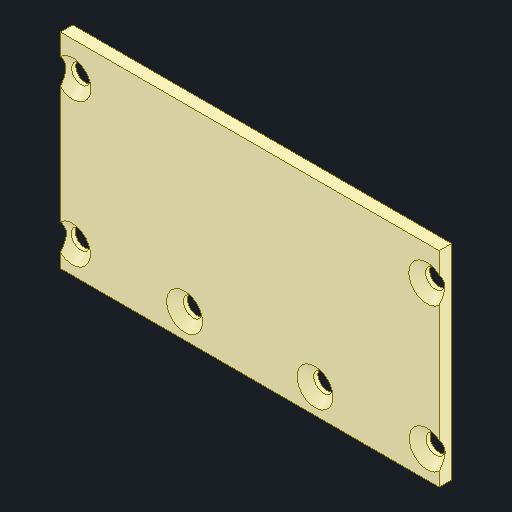
# Autodesk Inventor part: back
Saved by Autodesk Inventor 2023 (Build 270158000, 158)
## iProperties
Created: 2024-05-19
Part Number: back
Material: Nylon 6/6
Document SubType Name: Modeling
Designer: szymo
Density: 1.13 g/cm^3
Appearance: Nylon 6
Mass: 3.8512 g
Surface Area: 47.3773 cm^2
Volume: 3.40814 cm^3
Author: szymo
Autodesk Inventor part; units mm, degrees
ref_plane "YZ Plane" through (0, 0, 0) normal (1, 0, 0) x (0, 1, 0)
ref_plane "XZ Plane" through (0, 0, 0) normal (0, 1, 0) x (-1, 0, 0)
ref_plane "Work Plane1" through (22, 31.5, 0) normal (0, 0, 1) x (0, 1, 0)
sketch "Sketch1" plane through (22, 31.5, 0) normal (0, 0, 1) x (0, 1, 0)
  line L0 (0, 0) -> (0, 61) projected
  line L1 (0, 61) -> (-3.5, 61) projected
  line L2 (-3.5, 0) -> (-3.5, 61) projected
  circle A0 centre (-5.5, 2) radius 1.75 projected
  circle A1 centre (-28.5, 2) radius 1.75 projected
  line L3 (-3.5, 4) -> (-7.5, 4) projected
  arc A2 (-8.5, 3) -> (-7.5, 4) centre (-8.5, 4) ccw projected
  line L4 (-8.5, 3) -> (-21.7679, 3) projected
  arc A3 (-23.5, 4) -> (-21.7679, 3) centre (-21.7679, 5) ccw projected
  line L5 (-23.5, 4) -> (-31.5, 4) projected
  line L6 (-31.5, 0) -> (-31.5, 4) projected
  line L7 (-3.5, 0) -> (-3.5, 4) projected
  line L8 (-19.5, 22) -> (-3.5, 22) projected
  line L9 (-3.5, 22) -> (-3.5, 18) projected
  line L10 (-19.5, 39) -> (-3.5, 39) projected
  line L11 (-3.5, 39) -> (-3.5, 43) projected
  line L12 (-3.5, 57) -> (-6.7679, 57) projected
  line L13 (-3.5, 61) -> (-3.5, 57) projected
  line L14 (-3.5, 61) -> (-31.5, 61) projected
  line L15 (-31.5, 61) -> (-31.5, 57) projected
  line L16 (-24.004, 57) -> (-31.5, 57) projected
  line L17 (0, 0) -> (-32.9649, 0)
  line L18 (-32.9649, 0) -> (-32.9649, 61)
  line L19 (-32.9649, 61) -> (0, 61)
  line L20 (0, 61) -> (0, 0)
  line L21 (-3.5, 0) -> (-31.5, 0)
  line L22 (-8.5, 58) -> (-21.7679, 58) projected
  arc A4 (-7.634, 57.5) -> (-6.7679, 57) centre (-6.7679, 58) ccw projected
  arc A5 (-24.004, 57) -> (-23.2587, 57.3333) centre (-24.004, 58) ccw projected
  arc A6 (-21.7679, 58) -> (-23.2587, 57.3333) centre (-21.7679, 56) ccw projected
  arc A7 (-7.634, 57.5) -> (-8.5, 58) centre (-8.5, 57) ccw projected
  line L23 (-19.5, 18) -> (-19.5, 22) projected
  line L24 (-19.5, 18) -> (-3.5, 18) projected
  line L25 (-19.5, 43) -> (-3.5, 43) projected
  line L26 (-19.5, 43) -> (-19.5, 39) projected
  circle A8 centre (-5.5, 59) radius 1.75 projected
  circle A9 centre (-28.5, 59) radius 1.75 projected
  line L27 (-32.9649, 119.5) -> (-32.9649, -58.5) projected
  point P0 (-3.5, 28.5)
  point P1 (-3.5, 32.5)
  point P2 (-3.5, 61)
  point P3 (-13.5, 58)
  dimension "d25" = 0
  dimension "d26" = 0
  constraints: 10 end point, 1 collinear, 1 horizontal, 1 parallel, 1 perpendicular, 1 vertical, 1 other
  measures "d25" distance between parallel lines of L19 L1
  measures "d26" distance from line of point (-3.5, 0) L17
extrude "Extrusion1" add sketch "Sketch1" along normal blind 2 contours L17 L2 L1 L0 | L17 L6 L5 A3 L4 A2 L3 L2 | L2 L12 A4 A7 L22 A6 A5 L16 L15 L14 | L3 A2 L4 A3 L5 L6 L17 L18 L19 L15 L16 A5 A6 L22 A7 A4 L12 L2 L25 L26 L10 L8 L23 L24 | L24 L23 L8 L2 | L2 L10 L26 L25 | A0 | A1 | A8 | A9
hole "Hole1" at (20.0645, 2.9032, 2) at (20, 26, 2) at (2, 2.5, 2) at (-19, 2.5, 2) at (-37, 26, 2) at (-37.0645, 2.9032, 2) direction (0, 0, -1) diameter 3.1 end through all countersink diameter 5.8 countersink angle 90 clearance for "Countersunk Flat Head Screw ISO 2009/7046" size "M2.5" standard "ISO"
sketch "Sketch4" plane through (22, 31.5, 0) normal (0, 0, -1) x (-1, 0, 0)
  line L0 (39, -19.5) -> (39, -3.5)
  line L1 (39, -3.5) -> (43, -3.5)
  line L2 (43, -19.5) -> (43, -3.5)
  line L3 (43, -19.5) -> (39, -19.5)
  line L4 (22, -19.5) -> (22, -3.5)
  line L5 (18, -19.5) -> (22, -19.5)
  line L6 (18, -19.5) -> (18, -3.5)
  line L7 (22, -3.5) -> (18, -3.5)
  circle A0 centre (20, -29) radius 1.75
  line L8 (22, -31.5) -> (18, -31.5)
  line L9 (18, -31.5) -> (18, -19.5)
  line L10 (22, -19.5) -> (18, -19.5)
  line L11 (22, -19.5) -> (22, -31.5)
  circle A1 centre (41, -29) radius 1.75
  line L12 (39, -31.5) -> (43, -31.5)
  line L13 (39, -19.5) -> (39, -31.5)
  line L14 (39, -23.5) -> (43, -23.5)
  line L15 (43, -31.5) -> (43, -19.5)
  circle A2 centre (59, -5.5) radius 1.75
  circle A3 centre (59, -28.5) radius 1.75
  arc A4 (57, -6.7679) -> (57.5, -7.634) centre (58, -6.7679) ccw
  line L16 (57, -3.5) -> (57, -6.7679)
  line L17 (61, -3.5) -> (57, -3.5)
  line L18 (61, -3.5) -> (61, -31.5)
  line L19 (61, -31.5) -> (57, -31.5)
  line L20 (57, -24.004) -> (57, -31.5)
  arc A5 (57.3333, -23.2587) -> (57, -24.004) centre (58, -24.004) ccw
  arc A6 (57.3333, -23.2587) -> (58, -21.7679) centre (56, -21.7679) ccw
  line L21 (58, -8.5) -> (58, -21.7679)
  arc A7 (58, -8.5) -> (57.5, -7.634) centre (57, -8.5) ccw
  line L22 (61, -32.9649) -> (0, -32.9649)
  line L23 (0, -32.9649) -> (0, 0)
  line L24 (61, -32.9649) -> (0, -32.9649)
  line L25 (0, -32.9649) -> (0, -26.9649)
  line L26 (0, -26.9649) -> (61, -26.9649)
  line L27 (61, -26.9649) -> (61, -32.9649)
  line L28 (61, 0) -> (61, -32.9649)
  line L29 (0, -8.5) -> (61, -8.5)
  line L30 (61, -8.5) -> (61, -2.5)
  line L31 (61, -2.5) -> (0, -2.5)
  line L32 (0, -2.5) -> (0, -8.5)
  circle A8 centre (41, -29) radius 1.55
  line L33 (59, -5.5) -> (41, -29) construction
  line L34 (2, -5.5) -> (20, -29) construction
  circle A9 centre (41, -29) radius 2.9
  circle A10 centre (1.9355, -28.5968) radius 1.55
  line L35 (57, -26.9649) -> (57, -8.5)
  line L36 (4, -26.9649) -> (4, -8.5)
  line L37 (57, -10.5779) -> (44.4482, -26.9649)
  line L38 (54.8127, -8.5) -> (40.6693, -26.9649)
  line L39 (20.3307, -26.9649) -> (6.1873, -8.5)
  line L40 (4, -10.5779) -> (16.5518, -26.9649)
  circle A11 centre (20, -29) radius 2.9
  line L41 (61, -32.9649) -> (0, -32.9649)
  line L42 (0, -32.9649) -> (0, -30.7564)
  line L43 (0, 0) -> (61, 0)
  line L44 (61, 0) -> (61, -3.4)
  circle A12 centre (41, -29) radius 2.9
  arc A13 (61, -26.4372) -> (61, -30.7564) centre (59.0645, -28.5968) ccw
  arc A14 (0, -7.6) -> (0, -3.4) centre (2, -5.5) ccw
  arc A15 (0, -30.7564) -> (0, -26.4372) centre (1.9355, -28.5968) ccw
  arc A16 (61, -3.4) -> (61, -7.6) centre (59, -5.5) ccw
  line L45 (61, -7.6) -> (61, -26.4372)
  line L46 (61, -30.7564) -> (61, -32.9649)
  line L47 (0, -26.4372) -> (0, -7.6)
  line L48 (0, -3.4) -> (0, 0)
  line L49 (61, -3.5) -> (57, -3.5)
  line L50 (61, -3.5) -> (61, -31.5)
  line L51 (61, -31.5) -> (57, -31.5)
  line L52 (57, -3.5) -> (57, -31.5)
  line L53 (4, -26.9649) -> (18, -8.5) construction
  line L54 (57, -26.9649) -> (43, -8.5) construction
  line L55 (57, -24.4822) -> (44.8824, -8.5)
  line L56 (43, -10.9827) -> (55.1176, -26.9649)
  line L57 (5.8824, -26.9649) -> (18, -10.9827)
  line L58 (16.1176, -8.5) -> (4, -24.4822)
  circle A17 centre (41, -29) radius 1.55
  line L59 (22, -8.5) -> (41, -29) construction
  line L60 (39, -8.5) -> (20, -29) construction
  line L61 (39, -24.6355) -> (24.0452, -8.5)
  line L62 (22, -10.7066) -> (37.0687, -26.9649)
  line L63 (23.9313, -26.9649) -> (39, -10.7066)
  line L64 (36.9548, -8.5) -> (22, -24.6355)
  point P0 (42.4697, -31.5)
  point P1 (39.5303, -31.5)
  point P2 (18, -23.9221)
  point P3 (18, -8.5)
  point P4 (22, -8.5)
  point P5 (39, -8.5)
  point P6 (43, -23.9221)
  point P7 (0, -2.5)
  point P8 (28.4548, -17.6711)
  point P9 (30.5, -15.4644)
  point P10 (30.5, -19.8777)
  point P11 (49.8222, -15.0153)
  point P12 (47.9303, -17.4854)
  point P13 (57, -26.5602)
  point P14 (56.6672, -26.9649)
  point P15 (51.7021, -17.4946)
  point P16 (49.8101, -19.9647)
  point P17 (13.0697, -17.4854)
  point P18 (11.1778, -15.0153)
  point P19 (11.1899, -19.9647)
  point P20 (4.3328, -26.9649)
  point P21 (4, -26.5602)
  point P22 (9.2979, -17.4946)
  point P23 (32.5452, -17.6711)
extrude "zeberka" cut sketch "Sketch4" against normal blind 1 contours L13 L61 L63 L0 | L2 L56 L38 L15 | L64 L61 L29 | L62 L26 L63 | L29 L38 L55 | L64 L11 L4 L62 | L56 L26 L37 | L37 L35 L20 L55 | L6 L9 L39 L57 | L58 L39 L29 | L40 L26 L57 | L58 L36 L40
body "Solid1"
